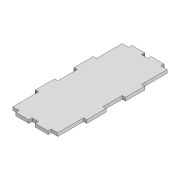
# Autodesk Inventor part: LAT 4
Saved by Autodesk Inventor 2022 (Build 260153000, 153)
## iProperties
Created: 2022-06-21
Part Number: LAT 4
Material: Generic
Document SubType Name: Modeling
Designer: ADMIN
Density: 1 g/cm^3
Appearance: Default
Author: ADMIN
Autodesk Inventor part; units mm, degrees
ref_plane "YZ Plane" through (0, 0, 0) normal (1, 0, 0) x (0, 1, 0)
ref_plane "XZ Plane" through (0, 0, 0) normal (0, 1, 0) x (-1, 0, 0)
ref_plane "XY Plane" through (0, 0, 0) normal (0, 0, 1) x (1, 0, 0)
sketch "Sketch1" plane through (0, 0, 0) normal (0, 1, 0) x (-1, 0, 0)
  line L0 (-65.5034, 14.4772) -> (4.4966, 14.4772)
  line L1 (4.4966, 14.4772) -> (4.4966, -155.5228)
  line L2 (4.4966, -155.5228) -> (-65.5034, -155.5228)
  line L3 (-65.5034, -155.5228) -> (-65.5034, 14.4772)
  line L4 (4.4966, -70.5228) -> (-65.5034, -70.5228) construction
  line L5 (-30.5034, 14.4772) -> (-30.5034, -155.5228) construction
  line L6 (4.4966, -25.5228) -> (9.4966, -25.5228)
  line L7 (9.4966, -25.5228) -> (9.4966, -55.5228)
  line L8 (9.4966, -55.5228) -> (4.4966, -55.5228)
  line L9 (4.4966, -55.5228) -> (4.4966, -25.5228)
  line L10 (4.4966, -85.5228) -> (9.4966, -85.5228)
  line L11 (9.4966, -85.5228) -> (9.4966, -115.5228)
  line L12 (9.4966, -115.5228) -> (4.4966, -115.5228)
  line L13 (4.4966, -115.5228) -> (4.4966, -85.5228)
  line L14 (-5.5034, 14.4772) -> (-25.5034, 14.4772)
  line L15 (-25.5034, 14.4772) -> (-25.5034, 19.4772)
  line L16 (-25.5034, 19.4772) -> (-5.5034, 19.4772)
  line L17 (-5.5034, 19.4772) -> (-5.5034, 14.4772)
  line L18 (-55.5034, 14.4772) -> (-35.5034, 14.4772)
  line L19 (-35.5034, 14.4772) -> (-35.5034, 19.4772)
  line L20 (-35.5034, 19.4772) -> (-55.5034, 19.4772)
  line L21 (-55.5034, 19.4772) -> (-55.5034, 14.4772)
  line L22 (-65.5034, -25.5228) -> (-70.5034, -25.5228)
  line L23 (-70.5034, -25.5228) -> (-70.5034, -55.5228)
  line L24 (-70.5034, -55.5228) -> (-65.5034, -55.5228)
  line L25 (-65.5034, -85.5228) -> (-70.5034, -85.5228)
  line L26 (-70.5034, -85.5228) -> (-70.5034, -115.5228)
  line L27 (-70.5034, -115.5228) -> (-65.5034, -115.5228)
  line L28 (-25.5034, -155.5228) -> (-25.5034, -160.5228)
  line L29 (-25.5034, -160.5228) -> (-5.5034, -160.5228)
  line L30 (-5.5034, -160.5228) -> (-5.5034, -155.5228)
  line L31 (-35.5034, -155.5228) -> (-35.5034, -160.5228)
  line L32 (-35.5034, -160.5228) -> (-55.5034, -160.5228)
  line L33 (-55.5034, -160.5228) -> (-55.5034, -155.5228)
  point P0 (0, 0)
  dimension "d0" = 170
  dimension "d1" = 70
  dimension "d2" = 5
  dimension "d3" = 30
  dimension "d4" = 5
  dimension "d5" = 30
  dimension "d6" = 30
  dimension "d7" = 15
  dimension "d8" = 20
  dimension "d9" = 20
  dimension "d10" = 5
  dimension "d11" = 5
  dimension "d12" = 10
  dimension "d13" = 5
  constraints: 68 end point, 16 symmetric about line, 10 parallel, 5 horizontal, 5 perpendicular, 4 midpoint, 4 point on line
  measures "d0" distance of L0.end L1.end
  measures "d1" distance of L1.end L2.end
  measures "d2" distance of L7.end L8.end
  measures "d3" distance of L6.end L7.end
  measures "d4" distance of L11.end L12.end
  measures "d5" distance of L10.end L11.end
  measures "d6" distance between parallel lines of L10 L8
  measures "d7" distance between parallel lines of L8 L4
  measures "d8" distance of L15.end L16.end
  measures "d9" distance of L20.end L19.end
  measures "d10" distance of L19.end L18.end
  measures "d11" distance of L16.end L14.start
  measures "d12" distance between parallel lines of L19 L15
  measures "d13" distance between parallel lines of L5 L19
extrude "Extrusion1" add sketch "Sketch1" along normal blind 5
body "Solid1"
